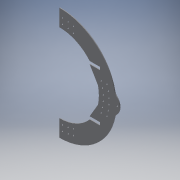
# Autodesk Inventor part: 19in outer coil TOP
Saved by Autodesk Inventor 2016 (Build 200138000, 138)
## iProperties
Created: 2016-01-31
Part Number: 19in outer coil TOP
Material: Copper, Alloy
Document SubType Name: Modeling
Designer: Scott
Density: 8.92 g/cm^3
Appearance: Copper - Satin
Mass: 1466.43 g
Surface Area: 1106.36 cm^2
Volume: 164.398 cm^3
Author: Scott
Autodesk Inventor part; units mm, degrees
ref_plane "YZ Plane" through (0, 0, 0) normal (1, 0, 0) x (0, 1, 0)
ref_plane "XZ Plane" through (0, 0, 0) normal (0, 1, 0) x (-1, 0, 0)
sketch "Sketch1" plane through (0, 0, 0) normal (0, 0, 1) x (1, 0, 0)
  circle A0 centre (62.4463, 65.7663) radius 3.175 projected
  circle A1 centre (37.8886, 72.253) radius 3.175 projected
  circle A2 centre (12.7, 75.5236) radius 3.175 projected
  circle A3 centre (12.7, 100.9706) radius 3.175 projected
  circle A4 centre (37.9341, 98.0724) radius 3.175 projected
  circle A5 centre (62.6728, 92.3141) radius 3.175 projected
  circle A6 centre (-62.6728, 92.3141) radius 3.175 projected
  circle A7 centre (-37.9341, 98.0724) radius 3.175 projected
  circle A8 centre (-12.7, 100.9706) radius 3.175 projected
  circle A9 centre (-12.7, 75.5236) radius 3.175 projected
  circle A10 centre (-37.8886, 72.253) radius 3.175 projected
  circle A11 centre (-62.4463, 65.7663) radius 3.175 projected
  circle A12 centre (-196.4399, -108.2163) radius 3.175 projected
  circle A13 centre (-193.1693, -83.0277) radius 3.175 projected
  circle A14 centre (-186.6826, -58.47) radius 3.175 projected
  circle A15 centre (-213.2304, -58.2435) radius 3.175 projected
  circle A16 centre (-218.9887, -82.9822) radius 3.175 projected
  circle A17 centre (-221.8868, -108.2163) radius 3.175 projected
  circle A18 centre (196.4399, -108.2163) radius 3.175 projected
  circle A19 centre (193.1693, -83.0277) radius 3.175 projected
  circle A20 centre (186.6826, -58.47) radius 3.175 projected
  circle A21 centre (213.2304, -58.2435) radius 3.175 projected
  circle A22 centre (218.9887, -82.9822) radius 3.175 projected
  circle A23 centre (221.8868, -108.2163) radius 3.175 projected
  arc A24 (241.3, -120.9163) -> (-241.3, -120.9163) centre (0, -120.9163) ccw projected
  line L0 (-241.3, -120.9163) -> (-177.8, -120.9163) projected
  arc A25 (177.8, -120.9163) -> (-177.8, -120.9163) centre (0, -120.9163) ccw projected
  line L1 (177.8, -120.9163) -> (241.3, -120.9163) projected
  circle A26 centre (-62.4463, -307.5989) radius 3.175 projected
  circle A27 centre (-37.8886, -314.0856) radius 3.175 projected
  circle A28 centre (-12.7, -317.3562) radius 3.175 projected
  circle A29 centre (-12.7, -342.8031) radius 3.175 projected
  circle A30 centre (-37.9341, -339.905) radius 3.175 projected
  circle A31 centre (-62.6728, -334.1466) radius 3.175 projected
  circle A32 centre (62.6728, -334.1466) radius 3.175 projected
  circle A33 centre (37.9341, -339.905) radius 3.175 projected
  circle A34 centre (12.7, -342.8031) radius 3.175 projected
  circle A35 centre (12.7, -317.3562) radius 3.175 projected
  circle A36 centre (37.8886, -314.0856) radius 3.175 projected
  circle A37 centre (62.4463, -307.5989) radius 3.175 projected
  circle A38 centre (196.4399, -133.6163) radius 3.175 projected
  circle A39 centre (193.1693, -158.8048) radius 3.175 projected
  circle A40 centre (186.6826, -183.3626) radius 3.175 projected
  circle A41 centre (213.2304, -183.5891) radius 3.175 projected
  circle A42 centre (218.9887, -158.8504) radius 3.175 projected
  circle A43 centre (221.8868, -133.6163) radius 3.175 projected
  circle A44 centre (-196.4399, -133.6163) radius 3.175 projected
  circle A45 centre (-193.1693, -158.8048) radius 3.175 projected
  circle A46 centre (-186.6826, -183.3626) radius 3.175 projected
  circle A47 centre (-213.2304, -183.5891) radius 3.175 projected
  circle A48 centre (-218.9887, -158.8504) radius 3.175 projected
  circle A49 centre (-221.8868, -133.6163) radius 3.175 projected
  arc A50 (-241.3, -120.9163) -> (241.3, -120.9163) centre (0, -120.9163) ccw projected
  line L2 (241.3, -120.9163) -> (177.8, -120.9163) projected
  arc A51 (-177.8, -120.9163) -> (177.8, -120.9163) centre (0, -120.9163) ccw projected
  line L3 (-177.8, -120.9163) -> (-241.3, -120.9163) projected
  circle A52 centre (0, -120.9163) radius 254
  line L4 (-254, -120.9163) -> (-254, 133.0837)
  line L5 (0, 133.0837) -> (-254, 133.0837)
  line L6 (-254, 100.9706) -> (-254, 104.1456)
  line L7 (-254, 56.8837) -> (-254, 60.0587)
  line L8 (0, -120.9163) -> (-254, 133.0837)
  line L9 (-179.6051, 58.6888) -> (-254, 133.0837)
  circle A53 centre (-216.8026, 95.8863) radius 3.302
  circle A54 centre (259.6856, -120.9163) radius 3.302
  arc A55 (271.0214, -121.5373) -> (259.974, -104.2042) centre (252.2597, -121.3082) ccw
  arc A56 (252.5671, -93.9743) -> (259.974, -104.2042) centre (265.1954, -92.6272) ccw
  line L10 (252.5671, -93.9743) -> (247.0534, -93.9743)
  line L11 (247.0534, -93.9743) -> (247.0534, -120.9163)
  arc A57 (257.0711, -139.4439) -> (271.0214, -121.5373) centre (252.2597, -121.3082) ccw
  arc A58 (257.0711, -139.4439) -> (252.5671, -147.8582) centre (265.1954, -149.2053) ccw
  line L12 (252.5671, -147.8582) -> (247.0534, -147.8582)
  line L13 (247.0534, -147.8582) -> (247.0534, -120.9163)
  line L14 (-254, -120.9163) -> (-254, -374.9163)
  line L15 (-254, -374.9163) -> (0, -374.9163)
  point P0 (0, 0)
  dimension "d0" = 508
  dimension "d3" = 6.604
  dimension "d7" = 6.604
  dimension "d8" = 12.7
  constraints: 24 end point, 12 point on circle, 7 centre point, 3 point on line, 3 tangent, 2 horizontal, 1 coincident, 1 collinear, 1 midpoint, 1 perpendicular, 1 vertical
  measures "d0" diameter of A52
  measures "d3" diameter of A53
  measures "d7" diameter of A54
  measures "d8" radius of A56
extrude "Extrusion1" add sketch "Sketch1" along normal blind 3.175 contours L1 A25 L8 A24 | A50 L0 A51 L1 | L8 A25 L0 A24 | A52 L12 L13 L11 L10 | A52 A56 A55 A57 A58 | L10 L11 L13 L12 A52 | A52 L8 A53 L5 | L15 L14 A52 | A52 L4 L8 A53 | A53 L8 | L8 A53
sketch "Sketch2" plane through (0, 0, 3.175) normal (0, 0, 1) x (1, 0, 0)
  circle A0 centre (259.6856, -120.9163) radius 3.302 projected
  arc A1 (252.5671, -93.9743) -> (0, 133.0837) centre (0, -120.9163) ccw projected
  line L0 (0, 133.0837) -> (-254, 133.0837) projected
  line L1 (-254, 133.0837) -> (-254, -374.9163) projected
  line L2 (-254, -374.9163) -> (0, -374.9163) projected
  arc A2 (0, -374.9163) -> (252.5671, -147.8582) centre (0, -120.9163) ccw projected
  arc A3 (257.0711, -139.4439) -> (252.5671, -147.8582) centre (265.1954, -149.2053) ccw projected
  arc A4 (257.0711, -139.4439) -> (259.974, -104.2042) centre (252.2597, -121.3082) ccw projected
  arc A5 (252.5671, -93.9743) -> (259.974, -104.2042) centre (265.1954, -92.6272) ccw projected
  circle A6 centre (-62.4463, -307.5989) radius 3.175 projected
  circle A7 centre (-37.8886, -314.0856) radius 3.175 projected
  circle A8 centre (-12.7, -317.3562) radius 3.175 projected
  circle A9 centre (-12.7, -342.8031) radius 3.175 projected
  circle A10 centre (-37.9341, -339.905) radius 3.175 projected
  circle A11 centre (-62.6728, -334.1466) radius 3.175 projected
  circle A12 centre (62.6728, -334.1466) radius 3.175 projected
  circle A13 centre (37.9341, -339.905) radius 3.175 projected
  circle A14 centre (12.7, -342.8031) radius 3.175 projected
  circle A15 centre (12.7, -317.3562) radius 3.175 projected
  circle A16 centre (37.8886, -314.0856) radius 3.175 projected
  circle A17 centre (62.4463, -307.5989) radius 3.175 projected
  circle A18 centre (196.4399, -133.6163) radius 3.175 projected
  circle A19 centre (193.1693, -158.8048) radius 3.175 projected
  circle A20 centre (186.6826, -183.3626) radius 3.175 projected
  circle A21 centre (213.2304, -183.5891) radius 3.175 projected
  circle A22 centre (218.9887, -158.8504) radius 3.175 projected
  circle A23 centre (221.8868, -133.6163) radius 3.175 projected
  circle A24 centre (-196.4399, -133.6163) radius 3.175 projected
  circle A25 centre (-193.1693, -158.8048) radius 3.175 projected
  circle A26 centre (-186.6826, -183.3626) radius 3.175 projected
  circle A27 centre (-213.2304, -183.5891) radius 3.175 projected
  circle A28 centre (-218.9887, -158.8504) radius 3.175 projected
  circle A29 centre (-221.8868, -133.6163) radius 3.175 projected
  circle A30 centre (221.8868, -108.2163) radius 3.175 projected
  circle A31 centre (218.9887, -82.9822) radius 3.175 projected
  circle A32 centre (213.2304, -58.2435) radius 3.175 projected
  circle A33 centre (186.6826, -58.47) radius 3.175 projected
  circle A34 centre (193.1693, -83.0277) radius 3.175 projected
  circle A35 centre (196.4399, -108.2163) radius 3.175 projected
  circle A36 centre (-221.8868, -108.2163) radius 3.175 projected
  circle A37 centre (-218.9887, -82.9822) radius 3.175 projected
  circle A38 centre (-213.2304, -58.2435) radius 3.175 projected
  circle A39 centre (-186.6826, -58.47) radius 3.175 projected
  circle A40 centre (-193.1693, -83.0277) radius 3.175 projected
  circle A41 centre (-196.4399, -108.2163) radius 3.175 projected
  circle A42 centre (-62.4463, 65.7663) radius 3.175 projected
  circle A43 centre (-37.8886, 72.253) radius 3.175 projected
  circle A44 centre (-12.7, 75.5236) radius 3.175 projected
  circle A45 centre (-12.7, 100.9706) radius 3.175 projected
  circle A46 centre (-37.9341, 98.0724) radius 3.175 projected
  circle A47 centre (-62.6728, 92.3141) radius 3.175 projected
  circle A48 centre (62.6728, 92.3141) radius 3.175 projected
  circle A49 centre (37.9341, 98.0724) radius 3.175 projected
  circle A50 centre (12.7, 100.9706) radius 3.175 projected
  circle A51 centre (12.7, 75.5236) radius 3.175 projected
  circle A52 centre (37.8886, 72.253) radius 3.175 projected
  circle A53 centre (62.4463, 65.7663) radius 3.175 projected
  circle A54 centre (0, -120.9163) radius 177.8 projected
  line L3 (0, -120.9163) -> (-321.8066, -120.9163)
  line L4 (-321.8066, -120.9163) -> (-321.8066, -440.0394)
  line L5 (-321.8066, -440.0394) -> (0, -440.0394)
  line L6 (0, -440.0394) -> (0, -120.9163)
  line L7 (0, -120.9163) -> (-359.6849, -120.9163)
  line L8 (-359.6849, -120.9163) -> (-359.6849, 186.2685)
  line L9 (-359.6849, 186.2685) -> (0, 186.2685)
  line L10 (0, 186.2685) -> (0, -120.9163)
  point P0 (0, 0)
  constraints: 16 end point, 4 parallel, 2 horizontal, 2 perpendicular
extrude "Extrusion2" cut sketch "Sketch2" against normal blind 25.4 contours L10 A54 L3 L1 L0 | L0 L1 L3 L7 L8 L9 L10 | L10 L3 A54 | L3 A54 L6 L2 L1 | L1 L2 L6 L5 L4 L3 | L3 L6 A54
sketch "Sketch3" plane through (0, 0, 3.175) normal (0, 0, 1) x (1, 0, 0)
  line L0 (0, 133.0837) -> (0, 56.8837) projected
  arc A0 (0, -298.7163) -> (0, 56.8837) centre (0, -120.9163) ccw projected
  line L1 (0, -298.7163) -> (0, -374.9163) projected
  arc A1 (0, -374.9163) -> (252.5671, -147.8582) centre (0, -120.9163) ccw projected
  arc A2 (257.0711, -139.4439) -> (252.5671, -147.8582) centre (265.1954, -149.2053) ccw projected
  arc A3 (257.0711, -139.4439) -> (259.974, -104.2042) centre (252.2597, -121.3082) ccw projected
  arc A4 (252.5671, -93.9743) -> (259.974, -104.2042) centre (265.1954, -92.6272) ccw projected
  arc A5 (252.5671, -93.9743) -> (0, 133.0837) centre (0, -120.9163) ccw projected
  circle A6 centre (259.6856, -120.9163) radius 3.302 projected
  circle A7 centre (62.6728, -334.1466) radius 3.175 projected
  circle A8 centre (37.9341, -339.905) radius 3.175 projected
  circle A9 centre (12.7, -342.8031) radius 3.175 projected
  circle A10 centre (12.7, -317.3562) radius 3.175 projected
  circle A11 centre (37.8886, -314.0856) radius 3.175 projected
  circle A12 centre (62.4463, -307.5989) radius 3.175 projected
  circle A13 centre (196.4399, -133.6163) radius 3.175 projected
  circle A14 centre (193.1693, -158.8048) radius 3.175 projected
  circle A15 centre (186.6826, -183.3626) radius 3.175 projected
  circle A16 centre (213.2304, -183.5891) radius 3.175 projected
  circle A17 centre (218.9887, -158.8504) radius 3.175 projected
  circle A18 centre (221.8868, -133.6163) radius 3.175 projected
  circle A19 centre (221.8868, -108.2163) radius 3.175 projected
  circle A20 centre (218.9887, -82.9822) radius 3.175 projected
  circle A21 centre (213.2304, -58.2435) radius 3.175 projected
  circle A22 centre (186.6826, -58.47) radius 3.175 projected
  circle A23 centre (193.1693, -83.0277) radius 3.175 projected
  circle A24 centre (196.4399, -108.2163) radius 3.175 projected
  circle A25 centre (62.6728, 92.3141) radius 3.175 projected
  circle A26 centre (37.9341, 98.0724) radius 3.175 projected
  circle A27 centre (12.7, 100.9706) radius 3.175 projected
  circle A28 centre (12.7, 75.5236) radius 3.175 projected
  circle A29 centre (37.8886, 72.253) radius 3.175 projected
  circle A30 centre (62.4463, 65.7663) radius 3.175 projected
  line L2 (259.6856, -120.9163) -> (273.9072, -120.9163)
  arc A31 (252.5671, -93.9743) -> (0, 133.0837) centre (0, -120.9163) ccw projected
  arc A32 (272.2239, -120.9163) -> (256.4729, -84.338) centre (221.8757, -120.9163) ccw
  arc A33 (249.0244, -70.8876) -> (248.8079, -69.822) centre (0, -120.9163) ccw
  arc A34 (249.0244, -70.8876) -> (256.4729, -84.338) centre (273.9268, -65.8847) ccw
  arc A35 (256.4729, -157.4946) -> (272.2239, -120.9163) centre (221.8757, -120.9163) ccw
  arc A36 (256.4729, -157.4946) -> (249.0244, -170.945) centre (273.9268, -175.9478) ccw
  line L3 (249.0244, -70.8876) -> (249.0244, -170.945)
  point P0 (0, 0)
  dimension "d13" = 25.4
  constraints: 12 point on circle, 5 centre point, 4 end point, 3 symmetric about line, 2 tangent, 1 horizontal, 1 point on line, 1 vertical, 2 other
  measures "d13" radius of A34
extrude "Extrusion3" add sketch "Sketch3" against normal blind 3.175 contours A34 A32 L2 A3 A4 A5 | A5 A4 A3 A2 A1 L3 | A1 A2 A3 L2 A35 A36
sketch "Sketch4" plane through (0, 0, 3.175) normal (0, 0, 1) x (1, 0, 0)
  circle A0 centre (259.6856, -120.9163) radius 3.302 projected
  circle A1 centre (62.4463, 65.7663) radius 3.175 projected
  circle A2 centre (37.8886, 72.253) radius 3.175 projected
  circle A3 centre (12.7, 75.5236) radius 3.175 projected
  circle A4 centre (12.7, 100.9706) radius 3.175 projected
  circle A5 centre (37.9341, 98.0724) radius 3.175 projected
  circle A6 centre (62.6728, 92.3141) radius 3.175 projected
  circle A7 centre (196.4399, -108.2163) radius 3.175 projected
  circle A8 centre (193.1693, -83.0277) radius 3.175 projected
  circle A9 centre (186.6826, -58.47) radius 3.175 projected
  circle A10 centre (213.2304, -58.2435) radius 3.175 projected
  circle A11 centre (218.9887, -82.9822) radius 3.175 projected
  circle A12 centre (221.8868, -108.2163) radius 3.175 projected
  circle A13 centre (221.8868, -133.6163) radius 3.175 projected
  circle A14 centre (218.9887, -158.8504) radius 3.175 projected
  circle A15 centre (213.2304, -183.5891) radius 3.175 projected
  circle A16 centre (186.6826, -183.3626) radius 3.175 projected
  circle A17 centre (193.1693, -158.8048) radius 3.175 projected
  circle A18 centre (196.4399, -133.6163) radius 3.175 projected
  circle A19 centre (62.4463, -307.5989) radius 3.175 projected
  circle A20 centre (37.8886, -314.0856) radius 3.175 projected
  circle A21 centre (12.7, -317.3562) radius 3.175 projected
  circle A22 centre (12.7, -342.8031) radius 3.175 projected
  circle A23 centre (37.9341, -339.905) radius 3.175 projected
  circle A24 centre (62.6728, -334.1466) radius 3.175 projected
  arc A25 (256.4729, -157.4946) -> (249.0244, -170.945) centre (273.9268, -175.9478) ccw projected
  arc A26 (256.4729, -157.4946) -> (256.4729, -84.338) centre (221.8757, -120.9163) ccw projected
  arc A27 (249.0244, -70.8876) -> (256.4729, -84.338) centre (273.9268, -65.8847) ccw projected
  arc A28 (249.0244, -70.8876) -> (0, 133.0837) centre (0, -120.9163) ccw projected
  line L0 (0, 133.0837) -> (0, 56.8837) projected
  arc A29 (0, -298.7163) -> (0, 56.8837) centre (0, -120.9163) ccw projected
  line L1 (0, -298.7163) -> (0, -374.9163) projected
  arc A30 (0, -374.9163) -> (249.0244, -170.945) centre (0, -120.9163) ccw projected
  circle A31 centre (62.4463, 65.7663) radius 3.302
  circle A32 centre (62.6728, 92.3141) radius 3.302
  circle A33 centre (37.8886, 72.253) radius 3.302
  circle A34 centre (37.9341, 98.0724) radius 3.302
  circle A35 centre (12.7, 75.5236) radius 3.302
  circle A36 centre (12.7, 100.9706) radius 3.302
  circle A37 centre (213.2304, -58.2435) radius 3.302
  circle A38 centre (186.6826, -58.47) radius 3.302
  circle A39 centre (193.1693, -83.0277) radius 3.302
  circle A40 centre (218.9887, -82.9822) radius 3.302
  circle A41 centre (221.8868, -108.2163) radius 3.302
  circle A42 centre (196.4399, -108.2163) radius 3.302
  circle A43 centre (196.4399, -133.6163) radius 3.302
  circle A44 centre (221.8868, -133.6163) radius 3.302
  circle A45 centre (218.9887, -158.8504) radius 3.302
  circle A46 centre (193.1693, -158.8048) radius 3.302
  circle A47 centre (186.6826, -183.3626) radius 3.302
  circle A48 centre (213.2304, -183.5891) radius 3.302
  circle A49 centre (62.4463, -307.5989) radius 3.302
  circle A50 centre (62.6728, -334.1466) radius 3.302
  circle A51 centre (37.9341, -339.905) radius 3.302
  circle A52 centre (37.8886, -314.0856) radius 3.302
  circle A53 centre (12.7, -317.3562) radius 3.302
  circle A54 centre (12.7, -342.8031) radius 3.302
  point P0 (0, 0)
  dimension "d19" = 6.604
  dimension "d20" = 6.604
  dimension "d21" = 6.604
  dimension "d22" = 6.604
  dimension "d23" = 6.604
  dimension "d24" = 6.604
  dimension "d25" = 6.604
  dimension "d26" = 6.604
  dimension "d27" = 6.604
  dimension "d28" = 6.604
  dimension "d29" = 6.604
  dimension "d30" = 6.604
  dimension "d31" = 6.604
  dimension "d32" = 6.604
  dimension "d33" = 6.604
  dimension "d34" = 6.604
  dimension "d35" = 6.604
  dimension "d36" = 6.604
  dimension "d37" = 6.604
  dimension "d38" = 6.604
  dimension "d39" = 6.604
  dimension "d40" = 6.604
  dimension "d41" = 6.604
  dimension "d42" = 6.604
  constraints: 24 centre point, 24 coincident
  measures "d19" diameter of A36
  measures "d20" diameter of A35
  measures "d21" diameter of A33
  measures "d22" diameter of A34
  measures "d23" diameter of A32
  measures "d24" diameter of A31
  measures "d25" diameter of A37
  measures "d26" diameter of A40
  measures "d27" diameter of A38
  measures "d28" diameter of A39
  measures "d29" diameter of A42
  measures "d30" diameter of A41
  measures "d31" diameter of A44
  measures "d32" diameter of A43
  measures "d33" diameter of A46
  measures "d34" diameter of A45
  measures "d35" diameter of A47
  measures "d36" diameter of A48
  measures "d37" diameter of A49
  measures "d38" diameter of A50
  measures "d39" diameter of A51
  measures "d40" diameter of A52
  measures "d41" diameter of A54
  measures "d42" diameter of A53
extrude "Extrusion4" cut sketch "Sketch4" against normal blind 3.175 contours A1 | A2 | A3 | A4 | A5 | A6 | A7 | A8 | A9 | A10 | A11 | A12 | A13 | A14 | A15 | A16 | A17 | A18 | A19 | A20 | A21 | A22 | A23 | A24 | A31 | A32 | A33 | A34 | A35 | A36 | A37 | A38 | A39 | A40 | A41 | A42 | A43 | A44 | A45 | A46 | A47 | A48 | A49 | A50 | A51 | A52 | A53 | A54
ref_plane "Work Plane1" through (105.3078, -6.6163, 117.475) normal (0, 1, 0) x (0, 0, 1)
sketch "Sketch5" plane through (105.3078, -6.6163, 117.475) normal (0, 1, 0) x (0, 0, 1)
  arc A0 (215.9, -105.3078) -> (-215.9, -105.3078) centre (0, -105.3078) ccw projected
  line L0 (-208.5631, -49.5025) -> (-31.405, -40.0564)
  line L1 (-31.405, -40.0564) -> (0, 110.5922)
  point P0 (-117.475, -105.3078)
  constraints: 4 end point, 2 point on circle
extrude "Extrusion5" cut sketch "Sketch5" against normal blind 12.7
sketch "Sketch8" plane through (0, 0, 3.175) normal (0, 0, 1) x (1, 0, 0)
  line L0 (136.1923, -6.6163) -> (183.162, -6.6163) projected
  line L1 (183.162, -6.6163) -> (183.162, -19.3163) projected
  line L2 (183.162, -19.3163) -> (145.9119, -19.3163) projected
  arc A0 (0, -298.7163) -> (145.9119, -19.3163) centre (0, -120.9163) ccw projected
  line L3 (0, -298.7163) -> (0, -374.9163) projected
  arc A1 (0, -374.9163) -> (249.0244, -170.945) centre (0, -120.9163) ccw projected
  arc A2 (256.4729, -157.4946) -> (249.0244, -170.945) centre (273.9268, -175.9478) ccw projected
  arc A3 (256.4729, -157.4946) -> (256.4729, -84.338) centre (221.8757, -120.9163) ccw projected
  arc A4 (249.0244, -70.8876) -> (256.4729, -84.338) centre (273.9268, -65.8847) ccw projected
  arc A5 (249.0244, -70.8876) -> (0, 133.0837) centre (0, -120.9163) ccw projected
  line L4 (0, 133.0837) -> (0, 56.8837) projected
  arc A6 (136.1923, -6.6163) -> (0, 56.8837) centre (0, -120.9163) ccw projected
  circle A7 centre (259.6856, -120.9163) radius 3.302 projected
  circle A8 centre (12.7, -342.8031) radius 3.302 projected
  circle A9 centre (37.8886, -314.0856) radius 3.302 projected
  circle A10 centre (62.6728, -334.1466) radius 3.302 projected
  circle A11 centre (213.2304, -183.5891) radius 3.302 projected
  circle A12 centre (193.1693, -158.8048) radius 3.302 projected
  circle A13 centre (221.8868, -133.6163) radius 3.302 projected
  circle A14 centre (196.4399, -108.2163) radius 3.302 projected
  circle A15 centre (218.9887, -82.9822) radius 3.302 projected
  circle A16 centre (186.6826, -58.47) radius 3.302 projected
  circle A17 centre (12.7, 100.9706) radius 3.302 projected
  circle A18 centre (37.9341, 98.0724) radius 3.302 projected
  circle A19 centre (62.6728, 92.3141) radius 3.302 projected
  circle A20 centre (62.4463, 65.7663) radius 3.302 projected
  circle A21 centre (37.8886, 72.253) radius 3.302 projected
  circle A22 centre (12.7, 75.5236) radius 3.302 projected
  circle A23 centre (213.2304, -58.2435) radius 3.302 projected
  circle A24 centre (193.1693, -83.0277) radius 3.302 projected
  circle A25 centre (221.8868, -108.2163) radius 3.302 projected
  circle A26 centre (196.4399, -133.6163) radius 3.302 projected
  circle A27 centre (218.9887, -158.8504) radius 3.302 projected
  circle A28 centre (186.6826, -183.3626) radius 3.302 projected
  circle A29 centre (62.4463, -307.5989) radius 3.302 projected
  circle A30 centre (37.9341, -339.905) radius 3.302 projected
  circle A31 centre (12.7, -317.3562) radius 3.302 projected
  line L5 (181.142, -19.3163) -> (181.142, -6.6163) projected
  line L6 (136.1923, -6.6163) -> (183.162, -6.6163) projected
  line L7 (183.162, -6.6163) -> (116.6118, -6.6163)
  line L8 (116.6118, -6.6163) -> (116.6118, -19.3163)
  line L9 (116.6118, -19.3163) -> (183.162, -19.3163)
  line L10 (183.162, -19.3163) -> (183.162, -6.6163)
  line L11 (259.6856, -120.9163) -> (145.9119, -120.9163)
  line L12 (183.162, -235.2163) -> (116.6118, -235.2163)
  line L13 (116.6118, -222.5163) -> (183.162, -222.5163)
  line L14 (183.162, -222.5163) -> (113.9696, -222.5163)
  line L15 (113.9696, -222.5163) -> (113.9696, -235.2163)
  line L16 (113.9696, -235.2163) -> (183.162, -235.2163)
  line L17 (183.162, -235.2163) -> (183.162, -222.5163)
  point P0 (0, 0)
  constraints: 22 end point, 4 parallel, 4 symmetric about line, 3 horizontal, 2 perpendicular
extrude "Extrusion6" cut sketch "Sketch8" against normal blind 25.4 contours L0 L5 L2 L9 L8 L7 | L0 L1 L2 L5 | L13 L17 L12 A0 | A0 L12 L16 L15 L14 L13
sketch "Sketch9" plane through (0, 0, 0) normal (0, 0, -1) x (-1, 0, 0)
  line L0 (-183.162, -222.5163) -> (-145.9119, -222.5163) projected
  arc A0 (-145.9119, -19.3163) -> (-145.9119, -222.5163) centre (0, -120.9163) ccw projected
  line L1 (-145.9119, -19.3163) -> (-183.162, -19.3163) projected
  line L2 (-183.162, -19.3163) -> (-183.162, -6.6163) projected
  line L3 (-183.162, -6.6163) -> (-136.1923, -6.6163) projected
  arc A1 (0, 56.8837) -> (-136.1923, -6.6163) centre (0, -120.9163) ccw projected
  line L4 (0, 56.8837) -> (0, 133.0837) projected
  arc A2 (0, 133.0837) -> (-249.0244, -70.8876) centre (0, -120.9163) ccw projected
  arc A3 (-256.4729, -84.338) -> (-249.0244, -70.8876) centre (-273.9268, -65.8847) ccw projected
  arc A4 (-256.4729, -84.338) -> (-256.4729, -157.4946) centre (-221.8757, -120.9163) ccw projected
  arc A5 (-249.0244, -170.945) -> (-256.4729, -157.4946) centre (-273.9268, -175.9478) ccw projected
  arc A6 (-249.0244, -170.945) -> (0, -374.9163) centre (0, -120.9163) ccw projected
  line L5 (0, -374.9163) -> (0, -298.7163) projected
  arc A7 (-136.1923, -235.2163) -> (0, -298.7163) centre (0, -120.9163) ccw projected
  line L6 (-136.1923, -235.2163) -> (-183.162, -235.2163) projected
  line L7 (-183.162, -235.2163) -> (-183.162, -222.5163) projected
  circle A8 centre (-12.7, -317.3562) radius 3.302 projected
  circle A9 centre (-37.9341, -339.905) radius 3.302 projected
  circle A10 centre (-62.4463, -307.5989) radius 3.302 projected
  circle A11 centre (-186.6826, -183.3626) radius 3.302 projected
  circle A12 centre (-218.9887, -158.8504) radius 3.302 projected
  circle A13 centre (-196.4399, -133.6163) radius 3.302 projected
  circle A14 centre (-221.8868, -108.2163) radius 3.302 projected
  circle A15 centre (-193.1693, -83.0277) radius 3.302 projected
  circle A16 centre (-213.2304, -58.2435) radius 3.302 projected
  circle A17 centre (-12.7, 75.5236) radius 3.302 projected
  circle A18 centre (-37.8886, 72.253) radius 3.302 projected
  circle A19 centre (-62.4463, 65.7663) radius 3.302 projected
  circle A20 centre (-62.6728, 92.3141) radius 3.302 projected
  circle A21 centre (-37.9341, 98.0724) radius 3.302 projected
  circle A22 centre (-12.7, 100.9706) radius 3.302 projected
  circle A23 centre (-186.6826, -58.47) radius 3.302 projected
  circle A24 centre (-218.9887, -82.9822) radius 3.302 projected
  circle A25 centre (-196.4399, -108.2163) radius 3.302 projected
  circle A26 centre (-221.8868, -133.6163) radius 3.302 projected
  circle A27 centre (-193.1693, -158.8048) radius 3.302 projected
  circle A28 centre (-213.2304, -183.5891) radius 3.302 projected
  circle A29 centre (-62.6728, -334.1466) radius 3.302 projected
  circle A30 centre (-37.8886, -314.0856) radius 3.302 projected
  circle A31 centre (-12.7, -342.8031) radius 3.302 projected
  circle A32 centre (-259.6856, -120.9163) radius 3.302 projected
  line L8 (-141.3083, -222.5163) -> (0, -222.5163) projected
  line L9 (-141.3083, -19.3163) -> (0, -19.3163) projected
  line L10 (-136.1923, -235.2163) -> (-136.1923, -222.5163) construction
  line L11 (-136.1923, -6.6163) -> (-183.162, -6.6163) projected
  line L12 (-136.1923, -6.6163) -> (-136.1923, -19.3163) construction
  line L13 (-145.9119, -222.5163) -> (-136.1923, -222.5163)
  line L14 (-145.9119, -19.3163) -> (-136.1923, -19.3163)
  line L15 (-136.1923, -222.5163) -> (-173.6699, -159.0163)
  arc A33 (-145.9119, -19.3163) -> (-145.9119, -222.5163) centre (0, -120.9163) ccw projected
  line L16 (-136.1923, -19.3163) -> (-173.6699, -82.8163)
  arc A34 (-173.6699, -159.0163) -> (-145.9119, -222.5163) centre (0, -120.9163) ccw
  line L17 (-183.162, -19.3163) -> (-145.9119, -19.3163) projected
  arc A35 (-145.9119, -19.3163) -> (-173.6699, -82.8163) centre (0, -120.9163) ccw
  point P0 (0, 0)
  dimension "d49" = 63.5
  dimension "d50" = 63.5
  constraints: 12 end point, 8 point on circle, 3 point on line, 2 centre point, 2 perpendicular, 1 parallel
  measures "d49" vertical distance of L10.end L15.end
  measures "d50" vertical distance of L12.end L16.end
extrude "Extrusion7" add sketch "Sketch9" against normal blind 3.175 contours A0 L15 L8 L13 | A0 L14 L9 L16
body "Solid1"
